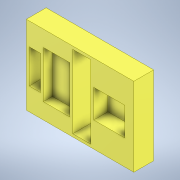
# Autodesk Inventor part: poeAdapter
Saved by Autodesk Inventor 2022.1 (Build 261234000, 234)
## iProperties
Created: 2021-08-20
Part Number: poeAdapter
Material: PC/ABS Plastic
Document SubType Name: Modeling
Designer: robst
Density: 0.357273 g/cm^3
Appearance: Smooth - Yellow
Author: robst
Autodesk Inventor part; units mm, degrees
ref_plane "YZ Plane" through (0, 0, 0) normal (1, 0, 0) x (0, 1, 0)
ref_plane "XZ Plane" through (0, 0, 0) normal (0, 1, 0) x (-1, 0, 0)
ref_plane "XY Plane" through (0, 0, 0) normal (0, 0, 1) x (1, 0, 0)
sketch "Sketch1" plane through (0, 0, 0) normal (0, 0, 1) x (1, 0, 0)
  line L0 (-94.85, -69.5) -> (94.85, -69.5)
  line L1 (94.85, -69.5) -> (94.85, 69.5)
  line L2 (94.85, 69.5) -> (-94.85, 69.5)
  line L3 (-94.85, 69.5) -> (-94.85, -69.5)
  line L4 (-94.85, -69.5) -> (94.85, 69.5) construction
  line L5 (94.85, -69.5) -> (-94.85, 69.5) construction
  point P0 (0, 0)
  dimension "d0" = 189.7
  dimension "d1" = 139
  constraints: 12 end point, 2 midpoint, 2 parallel, 1 horizontal, 1 perpendicular
  measures "d0" distance of L0.start L0.end
  measures "d1" distance of L1.end L0.end
extrude "MainBodyExtrusion" add sketch "Sketch1" against normal blind 35
sketch "Sketch3" plane through (0, 0, 0) normal (0, 0, 1) x (1, 0, 0)
  line L0 (24.15, -25) -> (79.15, -25)
  line L1 (79.15, -25) -> (79.15, 25)
  line L2 (79.15, 25) -> (24.15, 25)
  line L3 (24.15, 25) -> (24.15, -25)
  line L4 (24.15, -25) -> (79.15, 25) construction
  line L5 (79.15, -25) -> (24.15, 25) construction
  line L6 (94.85, -69.5) -> (94.85, 69.5) projected
  line L7 (0, 0) -> (94.85, 0) construction
  line L8 (-94.85, -69.5) -> (-94.85, 69.5) construction
  line L9 (-94.85, 69.5) -> (-94.85, -69.5) projected
  point P0 (51.65, 0)
  point P1 (51.65, 0)
  dimension "d5" = 15.7
  dimension "d6" = 50
  dimension "d7" = 55
  constraints: 14 end point, 4 midpoint, 2 parallel, 1 horizontal, 1 perpendicular, 1 point on line
  measures "d5" distance between parallel lines of L1 L6
  measures "d6" distance of L0.end L1.end
  measures "d7" distance of L1.end L2.end
extrude "HoleForCamera" cut sketch "Sketch3" against normal blind 25
sketch "Sketch4" plane through (0, 0, 0) normal (0, 0, 1) x (1, 0, 0)
  line L0 (0, 0) -> (-94.85, 0) construction
  line L1 (-94.85, -69.5) -> (-94.85, 69.5) construction
  line L2 (-89.85, -30) -> (-69.85, -30)
  line L3 (-69.85, -30) -> (-69.85, 30)
  line L4 (-69.85, 30) -> (-89.85, 30)
  line L5 (-89.85, 30) -> (-89.85, -30)
  line L6 (-89.85, -30) -> (-69.85, 30) construction
  line L7 (-69.85, -30) -> (-89.85, 30) construction
  point P0 (-79.85, 0)
  dimension "d13" = 20
  dimension "d14" = 60
  dimension "d15" = 5
  constraints: 14 end point, 3 midpoint, 2 parallel, 1 perpendicular, 1 point on line
  measures "d13" distance of L2.start L2.end
  measures "d14" distance of L3.end L2.end
  measures "d15" distance between parallel lines of L1 L5
extrude "HoleForFan" cut sketch "Sketch4" against normal blind 25
sketch "Sketch6" plane through (0, 0, 0) normal (0, 0, 1) x (1, 0, 0)
  line L0 (-94.85, -69.5) -> (-94.85, 69.5) construction
  line L1 (-94.85, 0) -> (94.85, 0) construction
  line L2 (94.85, 69.5) -> (94.85, -69.5) construction
  line L3 (-12.85, -64.5) -> (19.15, -64.5)
  line L4 (19.15, -64.5) -> (19.15, 64.5)
  line L5 (19.15, 64.5) -> (-12.85, 64.5)
  line L6 (-12.85, 64.5) -> (-12.85, -64.5)
  line L7 (-12.85, -64.5) -> (19.15, 64.5) construction
  line L8 (19.15, -64.5) -> (-12.85, 64.5) construction
  line L9 (24.15, -25) -> (24.15, 25) projected
  point P0 (0, 0)
  point P1 (3.15, 0)
  dimension "d20" = 32
  dimension "d21" = 129
  dimension "d24" = 5
  constraints: 14 end point, 4 midpoint, 3 parallel, 1 perpendicular, 1 point on line
  measures "d20" distance of L3.start L3.end
  measures "d21" distance of L4.end L3.end
  measures "d24" distance between parallel lines of L4 L9
extrude "HoleForPi" cut sketch "Sketch6" against normal blind 32.5
sketch "Sketch7" plane through (0, 0, 0) normal (0, 0, 1) x (1, 0, 0)
  line L0 (0, 0) -> (-94.85, 0) construction
  line L1 (-94.85, 69.5) -> (-94.85, -69.5) construction
  line L2 (-64.85, -41.5) -> (-17.85, -41.5)
  line L3 (-17.85, -41.5) -> (-17.85, 41.5)
  line L4 (-17.85, 41.5) -> (-64.85, 41.5)
  line L5 (-64.85, 41.5) -> (-64.85, -41.5)
  line L6 (-64.85, -41.5) -> (-17.85, 41.5) construction
  line L7 (-17.85, -41.5) -> (-64.85, 41.5) construction
  line L8 (-12.85, -64.5) -> (-12.85, 64.5) projected
  line L9 (-69.85, 30) -> (-69.85, -30) projected
  point P0 (-41.35, 0)
  dimension "d25" = 5
  dimension "d26" = 47
  dimension "d27" = 83
  dimension "d30" = 5
  constraints: 14 end point, 3 midpoint, 2 parallel, 1 perpendicular, 1 point on line
  measures "d25" distance between parallel lines of L3 L8
  measures "d26" distance of L2.start L2.end
  measures "d27" distance of L4.end L2.start
  measures "d30" distance between parallel lines of L9 L5
extrude "HoleForPoeAdapter" cut sketch "Sketch7" against normal blind 16
equation "\"d0\" = caseLength"
equation "\"d1\" = caseWidth"
equation "\"d2\" = oneHalfCaseDepth"
equation "\"d6\" = cameraWidth"
equation "\"d7\" = cameraLength"
equation "\"d8\" = 0.5 * cameraDepth"
equation "\"d13\" = fanDepth"
equation "\"d14\" = fanWidth"
equation "\"d15\" = wallThickness"
equation "\"d16\" = 0.5 * cameraDepth"
equation "\"d20\" = piCaseDepth"
equation "\"d21\" = piCaseLength"
equation "\"d22\" = 0.5 * piCaseWidth"
equation "\"d26\" = poeWidth"
equation "\"d27\" = poeLength"
equation "\"d28\" = 0.5 * piCaseDepth"
equation "\"fanWidth\" = 60"
equation "\"fanDepth\" = 20"
equation "\"wallThickness\" = 5"
equation "\"caseWidth\" = piCaseLength + 2 * wallThickness"
equation "\"cameraWidth\" = 50"
equation "\"oneHalfCaseDepth\" = 0.5 * fanWidth + wallThickness"
equation "\"caseLength\" = 189.7"
equation "\"cameraLength\" = 55"
equation "\"lensLength\" = 15.7"
equation "\"piCaseWidth\" = 65"
equation "\"piCaseDepth\" = 32"
equation "\"poeLength\" = 83"
equation "\"poeWidth\" = 47"
equation "\"poeDepth\" = 38"
equation "\"piEthernetCableReliefLength\" = 35"
equation "\"cameraDepth\" = 50"
equation "\"piCaseLength\" = 129"
body "Solid1"
